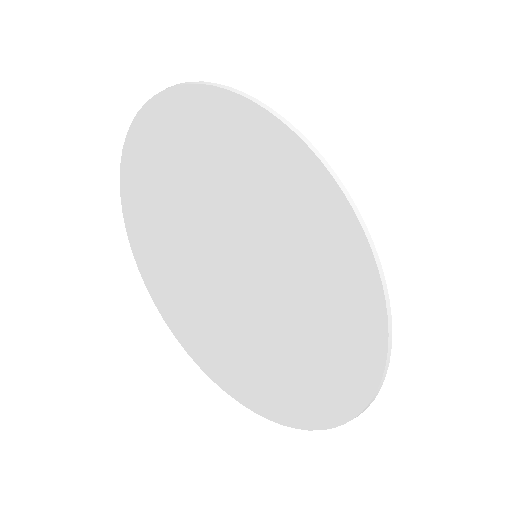
# Autodesk Inventor part: BUY - Cover glass - D12 x 0.17
Saved by Autodesk Inventor 2025.3 (Build 293356000, 356)
## iProperties
Part Number: BUY - Cover glass - D12 x 0.17
Material: Generic
Description: Round cover glass D12 mm, 0.17 mm
Document SubType Name: Modeling
Designer: benir
Appearance: Clear - Light
Author: benir
Autodesk Inventor part; units mm, degrees
ref_plane "YZ Plane" through (0, 0, 0) normal (1, 0, 0) x (0, 1, 0)
ref_plane "XZ Plane" through (0, 0, 0) normal (0, 1, 0) x (-1, 0, 0)
ref_plane "XY Plane" through (0, 0, 0) normal (0, 0, 1) x (1, 0, 0)
sketch "glass sketch" plane through (0, 0, 0) normal (0, 0, 1) x (1, 0, 0)
  circle A0 centre (0, 0) radius 6
  dimension "d0" = 12
  constraints: 1 centre point
  measures "d0" diameter of A0
extrude "glass" add sketch "glass sketch" along normal blind 0.17
equation "\"d0\" = glass_d"
equation "\"d1\" = glass_t"
equation "\"glass_d\" = 12"
equation "\"glass_t\" = 0.17"
body "Solid1"
